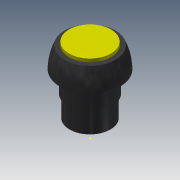
# Autodesk Inventor part: 800MR-D9D1
Saved by Autodesk Inventor 2015 (Build 190159000, 159)
## iProperties
Created: 2005-06-20
Part Number: 800MR-D9D1
Checked By: ~
Material: Delrin, Black
Document SubType Name: Modeling
Designer: BASSBW
Manufacturer: Standard
Standards Organization: Custom
Density: 1.425 g/cm^3
Appearance: Dark Gray
Description: PUSH BUTTON - MUSHROOM, NEMA 13
Vendor: AB
GlobalPropertyList: <PropertyList/>
SCALE: 1:1
STOCK SIZE: SEE DWG
UNITS: ANSI
COMMODITY: MFG
Author: BassBW
Autodesk Inventor part; units mm, degrees
ref_plane "YZ Plane" through (0, 0, 0) normal (1, 0, 0) x (0, 1, 0)
ref_plane "XZ Plane" through (0, 0, 0) normal (0, 1, 0) x (-1, 0, 0)
ref_plane "XY Plane" through (0, 0, 0) normal (0, 0, 1) x (1, 0, 0)
sketch "Sketch9" plane through (0, 0, 0) normal (0, 0, 1) x (1, 0, 0)
  line L0 (0, 0) -> (0, 10.5)
  line L1 (0, 0) -> (15, 0)
  arc A0 (15, 0) -> (12.7281, 10.5) centre (-10.4, 0) ccw
  line L2 (12.7281, 10.5) -> (0, 10.5)
  dimension "d35" = 30
  dimension "d37" = 25.4
  dimension "d43" = 10.5
  constraints: 6 end point, 2 perpendicular, 2 point on circle, 1 centre point, 1 point on line, 1 vertical
  measures "d35" diameter of L1.end L0
  measures "d37" radius of A0
  measures "d43" distance between parallel lines of L2 L1
revolve "Revolution1" add sketch "Sketch9" angle 360 about axis through (0, 0, 0) along (0, 1, 0)
sketch "Sketch10" plane through (0, 10.5, 0) normal (0, 1, 0) x (1, 0, 0)
  circle A0 centre (0, 0) radius 12.7281 projected
  circle A1 centre (0, 0) radius 10.5
  dimension "d39" = 21
  constraints: 1 centre point, 1 coincident
  measures "d39" diameter of A1
extrude "Extrusion6" add sketch "Sketch10" along normal blind 1.5875 contours A1
sketch "Sketch11" plane through (0, 0, 0) normal (0, -1, 0) x (1, 0, 0)
  circle A0 centre (0, 0) radius 15 projected
  circle A1 centre (0, 0) radius 11
  circle A2 centre (0, 0) radius 7.9375
  dimension "d42" = 22
  dimension "d44" = 15.875
  constraints: 2 centre point, 2 coincident
  measures "d42" diameter of A1
  measures "d44" diameter of A2
extrude "Extrusion7" add sketch "Sketch11" along normal blind 10.5 contours A1
sketch "Sketch12" plane through (0, -10.5, 0) normal (0, -1, 0) x (1, 0, 0)
  circle A0 centre (0, 0) radius 7.9375 projected
  circle A1 centre (0, 0) radius 11 projected
  circle A2 centre (0, 0) radius 10.2108
  dimension "d47" = 20.4216
  constraints: 1 centre point, 1 coincident
  measures "d47" diameter of A2
extrude "Extrusion8" add sketch "Sketch12" along normal blind 10.5 contours A2
sketch "Sketch13" plane through (0, -21, 0) normal (0, -1, 0) x (1, 0, 0)
  circle A0 centre (0, 0) radius 5.08
  point P0 (-5.08, 0)
  point P1 (5.08, 0)
  dimension "d52" = 10.16
  constraints: 2 point on circle, 1 centre point, 1 coincident
  measures "d52" diameter of A0
body "Solid1"
